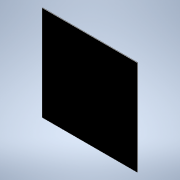
# Autodesk Inventor part: Black Construction Hardboard
Saved by Autodesk Inventor 2022.1 (Build 261234020, 234B)
## iProperties
Created: 2021-11-04
Part Number: Black Construction Hardboard
Material: Generic
Document SubType Name: Modeling
Designer: gnzak
Density: 1 g/cm^3
Appearance: Default
Author: gnzak
Autodesk Inventor part; units mm, degrees
ref_plane "YZ Plane" through (0, 0, 0) normal (1, 0, 0) x (0, 1, 0)
ref_plane "XZ Plane" through (0, 0, 0) normal (0, 1, 0) x (-1, 0, 0)
ref_plane "XY Plane" through (0, 0, 0) normal (0, 0, 1) x (1, 0, 0)
sketch "Sketch1" plane through (0, 0, 0) normal (0, 0, 1) x (1, 0, 0)
  line L0 (-363.22, 363.22) -> (363.22, 363.22)
  line L1 (363.22, 363.22) -> (363.22, -363.22)
  line L2 (363.22, -363.22) -> (-363.22, -363.22)
  line L3 (-363.22, -363.22) -> (-363.22, 363.22)
  point P0 (0, 0)
  dimension "d0" = 726.44
  dimension "d1" = 726.44
  dimension "d2" = 363.22
  dimension "d3" = 363.22
  constraints: 8 end point, 2 parallel, 1 horizontal, 1 perpendicular
  measures "d0" distance of L2.end L0.start
  measures "d1" distance of L0.start L0.end
  measures "d2" distance from line of point (0, 0) L3
  measures "d3" distance from line of point (0, 0) L0
extrude "Extrusion1" add sketch "Sketch1" along normal blind 4.7625
equation "\"d2\" = 0.5 * d1"
equation "\"d3\" = 0.5 * d0"
body "Solid1"
